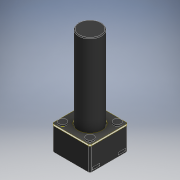
# Autodesk Inventor part: Button_üst
Saved by Autodesk Inventor 2021 (Build 250183000, 183)
## iProperties
Created: 2019-08-05
Part Number: Button_üst
Material: Rubber, Silicone
Document SubType Name: Modeling
Designer: Yusuf
Mass: 0.1078 g
Surface Area: 1.79163 cm^2
Volume: 0.0862402 cm^3
Density: 1.25 g/cm^3
Appearance: Rubber - Black
Author: Yusuf
Autodesk Inventor part; units mm, degrees
ref_plane "YZ Plane" through (0, 0, 0) normal (1, 0, 0) x (0, 1, 0)
ref_plane "XZ Plane" through (0, 0, 0) normal (0, 1, 0) x (-1, 0, 0)
sketch "Sketch1" plane through (0, 0, 0) normal (0, 1, 0) x (-1, 0, 0)
  line L0 (-2.5, -2.5) -> (2.5, -2.5)
  line L1 (2.5, -2.5) -> (2.5, 2.5)
  line L2 (2.5, 2.5) -> (-2.5, 2.5)
  line L3 (-2.5, 2.5) -> (-2.5, -2.5)
  line L4 (-2.5, -2.5) -> (2.5, 2.5) construction
  line L5 (2.5, -2.5) -> (-2.5, 2.5) construction
  point P0 (0, 0)
  dimension "d0" = 5
  dimension "d1" = 5
  constraints: 12 end point, 2 midpoint, 2 parallel, 1 horizontal, 1 perpendicular
  measures "d0" distance of L2.end L1.end
  measures "d1" distance of L1.end L0.end
extrude "Extrusion1" add sketch "Sketch1" along normal blind 3
sketch "Sketch2" plane through (0, 3, 0) normal (0, 1, 0) x (1, 0, 0)
  line L0 (-2.5, -2.5) -> (2.5, -2.5) projected
  line L1 (2.5, 2.5) -> (-2.5, 2.5)
  line L2 (-2.5, 2.5) -> (-2.5, -2.5)
  line L3 (-2.5, -2.5) -> (2.5, -2.5)
  line L4 (2.5, -2.5) -> (2.5, 2.5)
  line L5 (2.5, 2.5) -> (-2.5, -2.5) construction
  line L6 (-2.5, 2.5) -> (2.5, -2.5) construction
  circle A0 centre (0, 0) radius 1.6
  circle A1 centre (0, 0) radius 1.5
  dimension "d4" = 3.2
  dimension "d5" = 3
  constraints: 12 end point, 2 centre point, 2 coincident, 2 midpoint, 2 parallel, 1 horizontal, 1 perpendicular
  measures "d4" diameter of A0
  measures "d5" diameter of A1
extrude "Extrusion2" add sketch "Sketch2" along normal blind 11 contours A1
extrude "Extrusion3" add sketch "Sketch2" along normal blind 0.2 separate body contours L2 L1 L4 L0
sketch "Sketch3" plane through (0, 3.2, 0) normal (0, 1, 0) x (1, 0, 0)
  line L0 (-2.5, 2.5) -> (-2.5, -2.5) projected
  line L1 (2.5, 2.5) -> (-2.5, 2.5) projected
  line L2 (-2.5, -2.5) -> (2.5, 2.5) construction
  circle A0 centre (-1.8, -1.8) radius 0.5
  line L3 (-2.5, -2.5) -> (2.5, -2.5) projected
  line L4 (2.5, -2.5) -> (-2.5, 2.5) construction
  point P0 (0, 0)
  point P1 (-1.8, 1.8)
  point P2 (1.8, 1.8)
  point P3 (1.8, -1.8)
  dimension "d10" = 1
  dimension "d11" = 1.8
  constraints: 4 end point, 4 point on line, 1 centre point
  measures "d10" diameter of A0
  measures "d11" horizontal distance of point (0, 0) A0.centre
ref_plane "Work Plane1" through (-1.8, 3.2, 1.8) normal (0.7071068, 0, -0.7071068) x (0, 1, 0)
sketch "Sketch4" plane through (-1.8, 3.2, 1.8) normal (0.7071068, 0, -0.7071068) x (0, 1, 0)
  line L0 (0, -0.5) -> (0, 0.5) projected
  arc A0 (0.2, 0.5) -> (0, 0.5) centre (0.1, 0.3882) ccw
  line L1 (0, 0) -> (0.2, 0)
  line L2 (0.2, 0.5) -> (0.2, 0)
  line L3 (0, 0) -> (0, 0.5)
  point P0 (-3.2, 0)
  dimension "d12" = 0.2
  dimension "d13" = 0.15
  dimension "d14" = 0.1
  dimension "d17" = 0.2
  constraints: 6 end point, 2 point on circle, 1 centre point, 1 horizontal, 1 vertical
  measures "d12" distance of L0.end L2.start
  measures "d13" radius of A0
  measures "d14" distance from line of L0 A0.centre
  measures "d17" distance of L1.start L1.end
ref_plane "Work Plane2" through (-1.4464, 3.4, 2.1536) normal (0, 1, 0) x (1, 0, 0)
revolve "Revolution1" add sketch "Sketch4" angle 360 about axis through (-1.8, 3.2, 1.8) along (0, 1, 0) bodies 1
pattern_sketch "Sketch Driven Pattern1" of "Revolution1" from (-1.8, 3.2, 1.8) bodies 1 copies at (-1.8, 3.2, -1.8) at (1.8, 3.2, -1.8) at (1.8, 3.2, 1.8)
sketch "Sketch6" plane through (-2.5, 0, -2.5) normal (-1, 0, 0) x (0, 0, 1)
  line L0 (3.7, 0.5) -> (4.7, 0.5)
  line L1 (4.7, 0.5) -> (4.7, 0.2)
  line L2 (4.7, 0.2) -> (3.7, 0.2)
  line L3 (3.7, 0.2) -> (3.7, 0.5)
  line L4 (3.7, 0.5) -> (4.7, 0.2) construction
  line L5 (4.7, 0.5) -> (3.7, 0.2) construction
  line L6 (5, 0) -> (5, 3) projected
  line L7 (0, 0) -> (5, 0) projected
  point P0 (2.5, 0)
  point P1 (4.2, 0.35)
  dimension "d19" = 1
  dimension "d20" = 0.3
  dimension "d21" = 0.3
  dimension "d22" = 0.2
  constraints: 12 end point, 2 midpoint, 2 parallel, 1 horizontal, 1 perpendicular
  measures "d19" distance of L1.end L2.end
  measures "d20" distance of L0.end L1.end
  measures "d21" distance between parallel lines of L6 L1
  measures "d22" distance between parallel lines of L7 L2
extrude "Extrusion4" cut sketch "Sketch6" against normal blind 1 bodies 1
pattern_linear "Rectangular Pattern1" count 2 spacing 3.4 along (0, 0, -1) count 2 spacing 4 along (1, 0, 0) of "Extrusion4" bodies 1
fillet "Fillet1" radius 0.2 8 edges at (-2.5, 1.5, -2.5) (2.5, 1.5, -2.5) (-2.5, 1.5, 2.5) (2.5, 1.5, 2.5) (-2.5, 3.1, 2.5) (-2.5, 3.1, -2.5) (2.5, 3.1, -2.5) (2.5, 3.1, 2.5)
fillet "Fillet2" radius 0.1 1 edges at (-1.5, 14, 0)
body "Solid1"
body "Solid2"
